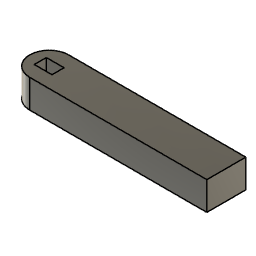
3DTegning_laase_arm v1 (Autodesk Fusion 360 design; units mm, degrees)
Autodesk Fusion 360 part; units mm, degrees
sketch "Sketch1" plane through (0, 0, 0) normal (0, 0, 1) x (1, 0, 0)
  line L0 (0, 0) -> (5, 0)
  line L1 (5, 0) -> (5, 3.4)
  line L2 (5, 3.4) -> (0, 3.4)
  line L3 (0, 3.4) -> (0, 0)
  circle A0 centre (2.5, 1.7) radius 5.5
  line L4 (2.5, -3.8) -> (52.5, -3.8)
  line L5 (2.5, 7.2) -> (52.5, 7.2)
  line L6 (52.5, 7.2) -> (52.5, -3.8)
  dimension "d1" = 5
  dimension "d2" = 3.4
  dimension "d3" = 5
  dimension "d4" = 11
  dimension "d5" = 50
  constraint coincident L0.start L3.end
  constraint horizontal L0
  constraint perpendicular L0 L1
  constraint perpendicular L1 L2
  constraint coincident A0 L4.start
  constraint perpendicular L1 L4
  constraint coincident A0 L5.start
  constraint tangent A0 L5
  constraint parallel L4 L5
  constraint perpendicular L4 L6
  measures "d1" distance of L0.start L0.end
  measures "d2" distance of L0.end L1.end
  measures "d3" distance of L1.end L2.end
  measures "d4" diameter of A0
  measures "d5" distance of L4.start L4.end
extrude "Extrude1" add sketch "Sketch1" along normal blind 6
extrude "Extrude2" add sketch "Sketch1" against normal blind 2 contours L0 L1 L2 L3 | A0 | A0 L4 L5 L6
